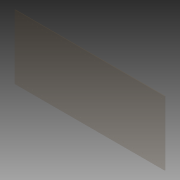
# Autodesk Inventor part: Front Screen
Saved by Autodesk Inventor 2012 (Build 160160000, 160)
## iProperties
Created: 2011-10-21
Part Number: Front Screen
Material: Polycarbonate, Smoke
Document SubType Name: Modeling
Designer: Ian Walters
Mass: 1045.29 g
Surface Area: 5559.67 cm^2
Volume: 871.075 cm^3
Density: 1.2 g/cm^3
Author: Ian Walters
Autodesk Inventor part; units mm, degrees
ref_plane "YZ Plane" through (0, 0, 0) normal (1, 0, 0) x (0, 1, 0)
ref_plane "XZ Plane" through (0, 0, 0) normal (0, 1, 0) x (-1, 0, 0)
ref_plane "XY Plane" through (0, 0, 0) normal (0, 0, 1) x (1, 0, 0)
sketch "Sketch1" plane through (0, 0, 0) normal (0, 0, 1) x (1, 0, 0)
  line L0 (-400.05, 171.45) -> (400.05, 171.45)
  line L1 (400.05, 171.45) -> (400.05, -171.45)
  line L2 (400.05, -171.45) -> (-400.05, -171.45)
  line L3 (-400.05, -171.45) -> (-400.05, 171.45)
  point P0 (0, 0)
  point P1 (0, 171.45)
  point P2 (400.05, 0)
  dimension "d0" = 800.1
  dimension "d1" = 342.9
  constraints: 8 end point, 2 midpoint, 2 parallel, 1 horizontal, 1 horizontal alignment, 1 perpendicular, 1 vertical alignment
  measures "d0" distance of L1.end L2.end
  measures "d1" distance of L0.end L1.end
extrude "Extrusion1" add sketch "Sketch1" along normal blind 3.175
sketch "Sketch2" plane through (0, 0, 3.175) normal (0, 0, 1) x (1, 0, 0)
  line L0 (-400.05, 171.45) -> (400.05, 171.45) projected
  line L1 (-400.05, -171.45) -> (-400.05, 171.45) projected
  line L2 (400.05, -171.45) -> (-400.05, -171.45) projected
  circle A0 centre (-381, 152.4) radius 2.3813
  line L3 (-400.05, 0) -> (0, 0) construction
  circle A1 centre (-381, -152.4) radius 2.3813
  dimension "d4" = 4.7625
  dimension "d5" = 19.05
  dimension "d6" = 19.05
  constraints: 2 centre point, 2 end point, 1 midpoint, 1 parallel, 1 symmetric about line, 1 other
  measures "d4" diameter of A0
  measures "d5" distance from line of L1 A0.centre
  measures "d6" distance from line of L0 A0.centre
extrude "Extrusion2" cut sketch "Sketch2" against normal up to next
pattern_linear "Rectangular Pattern1" count 31 spacing 25.4 along (1, 0, 0) of "Extrusion2"
equation "\"d6\" = d5"
body "Solid1"
